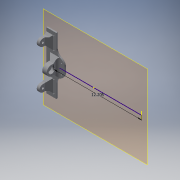
# Autodesk Inventor part: YEnd
Saved by Autodesk Inventor 2016 (Build 200138000, 138)
## iProperties
Created: 2016-04-23
Part Number: YEnd
Material: Generic
Document SubType Name: Modeling
Designer: Scott
Density: 1 g/cm^3
Appearance: Default
Author: Scott
Autodesk Inventor part; units mm, degrees
ref_plane "YZ Plane" through (0, 0, 0) normal (1, 0, 0) x (0, 1, 0)
ref_plane "XZ Plane" through (0, 0, 0) normal (0, 1, 0) x (-1, 0, 0)
ref_plane "XY Plane" through (0, 0, 0) normal (0, 0, 1) x (1, 0, 0)
ref_plane "Work Plane1" through (0, 0, 0) normal (0, 0, 1) x (1, 0, 0)
sketch "Sketch1" plane through (0, 0, 0) normal (0, 0, 1) x (1, 0, 0)
  circle A0 centre (-142.875, 44.45) radius 2.2225
  circle A1 centre (-142.875, 88.9) radius 2.2225
  circle A2 centre (-115.9342, 17.5092) radius 2.2225
  circle A3 centre (-115.9342, -17.5092) radius 2.2225
  circle A4 centre (-142.875, -44.45) radius 2.2225
  circle A5 centre (-142.875, -88.9) radius 2.2225
  line L0 (-168.275, 133.904) -> (-168.275, -133.904)
  line L1 (-103.6936, -28.7748) -> (-168.275, -28.7748)
  line L2 (-168.275, -28.7748) -> (-168.275, 28.7748)
  line L3 (-168.275, 28.7748) -> (-103.6936, 28.7748)
  line L4 (-103.6936, 28.7748) -> (-103.6936, -28.7748)
  line L5 (-103.6936, -28.7748) -> (-168.275, 28.7748) construction
  line L6 (-168.275, -28.7748) -> (-103.6936, 28.7748) construction
  line L7 (-133.3967, -101.2471) -> (-168.275, -101.2471)
  line L8 (-168.275, -101.2471) -> (-168.275, 101.2471)
  line L9 (-168.275, 101.2471) -> (-133.3967, 101.2471)
  line L10 (-133.3967, 101.2471) -> (-133.3967, -101.2471)
  line L11 (-133.3967, -101.2471) -> (-168.275, 101.2471) construction
  line L12 (-168.275, -101.2471) -> (-133.3967, 101.2471) construction
  point P0 (0, 0)
  point P1 (-135.9843, 0)
  point P2 (-150.8358, 0)
extrude "Extrusion1" add sketch "Sketch1" along normal blind 5.08
fillet "Fillet1" radius 25.4 4 edges at (-133.3967, 28.7748, 2.54) (-133.3967, -28.7748, 2.54) (-103.6936, 28.7748, 2.54) (-103.6936, -28.7748, 2.54)
sketch "Sketch2" plane through (0, 0, 5.08) normal (0, 0, 1) x (1, 0, 0)
  line L0 (168.275, 12.5) -> (168.275, -12.5) projected
  line L1 (168.275, 0) -> (-141.725, 0)
  point P0 (0, 0)
  dimension "d3" = 310
  constraints: 2 end point, 1 horizontal, 1 midpoint
  measures "d3" distance of L1.start L1.end
ref_plane "Work Plane2" through (-141.725, 0, 5.08) normal (-1, 0, 0) x (0, -1, 0)
sketch "Sketch3" plane through (-141.725, 0, 5.08) normal (-1, 0, 0) x (0, -1, 0)
  circle A0 centre (0, 21.59) radius 5 projected
  circle A1 centre (0, 21.59) radius 11 projected
  circle A2 centre (0, 21.59) radius 17.3577
  line L0 (-17.3577, 21.59) -> (-17.3577, 0)
  line L1 (-101.2471, 0) -> (101.2471, 0) projected
  line L2 (17.3577, 21.59) -> (17.3577, 0)
  circle A3 centre (-70, 21.59) radius 4 projected
  circle A4 centre (70, 21.59) radius 4 projected
  circle A5 centre (-70, 21.59) radius 12.7105
  circle A6 centre (70, 21.59) radius 12.7105
  line L3 (82.7105, 21.59) -> (82.7105, 0)
  line L4 (57.2895, 21.59) -> (57.2895, 0)
  line L5 (-57.2895, 21.59) -> (-57.2895, 0)
  line L6 (-82.7105, 21.59) -> (-82.7105, 0)
  line L7 (-82.7105, 0) -> (-57.2895, 0)
  line L8 (-17.3577, 0) -> (17.3577, 0)
  line L9 (57.2895, 0) -> (82.7105, 0)
  point P0 (0, -5.08)
  constraints: 18 end point, 6 perpendicular, 6 point on circle, 6 point on line, 5 tangent, 3 centre point, 3 coincident, 1 collinear, 1 parallel, 1 vertical
extrude "Extrusion2" add sketch "Sketch3" against normal up to surface (8.3283 mm away) contours A2 | L2 L1 L0 A2 | L6 A5 L5 L1 | A5 | L4 A6 L3 L1 | A6
sketch "Sketch4" plane through (-141.725, 0, 5.08) normal (-1, 0, 0) x (0, 0, 1)
  circle A0 centre (21.59, 70) radius 4 projected
  line L0 (0, 57.2895) -> (21.59, 57.2895) projected
  arc A1 (21.59, 57.2895) -> (21.59, 82.7105) centre (21.59, 70) ccw projected
  line L1 (21.59, 82.7105) -> (0, 82.7105) projected
  line L2 (0, 57.2895) -> (0, 82.7105) projected
  circle A2 centre (21.59, -70) radius 4 projected
  line L3 (0, -82.7105) -> (0, -57.2895) projected
  line L4 (0, -82.7105) -> (21.59, -82.7105) projected
  arc A3 (21.59, -82.7105) -> (21.59, -57.2895) centre (21.59, -70) ccw projected
  line L5 (21.59, -57.2895) -> (0, -57.2895) projected
  point P0 (-5.08, 0)
extrude "Extrusion3" add sketch "Sketch4" along normal blind 10.16
chamfer "Chamfer1" distance 14.2875 angle 45 2 edges at (-151.885, 70, 5.08) (-151.885, -70, 5.08)
sketch "Sketch5" plane through (-133.3967, -17.3577, 5.08) normal (1, 0, 0) x (0, 0, -1)
  line L0 (0, 34.7154) -> (0, 0) projected
  line L1 (-21.59, 34.7154) -> (0, 34.7154) projected
  arc A0 (-21.59, 34.7154) -> (-21.59, 0) centre (-21.59, 17.3577) ccw projected
  line L2 (0, 0) -> (-21.59, 0) projected
  circle A1 centre (-21.59, 17.3577) radius 11 projected
  circle A2 centre (-21.59, 17.3577) radius 5
  point P0 (5.08, 17.3577)
  dimension "d11" = 10
  constraints: 1 centre point, 1 coincident
  measures "d11" diameter of A2
extrude "Extrusion4" add sketch "Sketch5" along normal blind 5.08 contours L0 L2 A0 L1 | A1
fillet "Fillet2" radius 9.525 1 edges at (-128.3167, 0, 5.08)
chamfer "Chamfer2" distance 14.2875 angle 45 1 edges at (-141.725, 0, 5.08)
sketch "Sketch6" plane through (-133.3967, -101.2471, 5.08) normal (1, 0, 0) x (0, 0, -1)
  line L0 (0, 18.5366) -> (-14.2875, 18.5366) projected
  line L1 (-14.2875, 18.5366) -> (-14.2875, 43.9576) projected
  line L2 (-14.2875, 43.9576) -> (0, 43.9576) projected
  line L3 (0, 43.9576) -> (0, 18.5366) projected
  line L4 (-14.2875, 18.5366) -> (-14.2875, 43.9576) projected
  line L5 (-14.2875, 18.5366) -> (-21.59, 18.5366) projected
  arc A0 (-21.59, 43.9576) -> (-21.59, 18.5366) centre (-21.59, 31.2471) ccw projected
  line L6 (-21.59, 43.9576) -> (-14.2875, 43.9576) projected
  circle A1 centre (-21.59, 31.2471) radius 4 projected
  line L7 (-14.2875, 158.5366) -> (-14.2875, 183.9576) projected
  line L8 (-14.2875, 158.5366) -> (-21.59, 158.5366) projected
  arc A2 (-21.59, 183.9576) -> (-21.59, 158.5366) centre (-21.59, 171.2471) ccw projected
  line L9 (-21.59, 183.9576) -> (-14.2875, 183.9576) projected
  circle A3 centre (-21.59, 171.2471) radius 4 projected
  line L10 (0, 158.5366) -> (-14.2875, 158.5366) projected
  line L11 (-14.2875, 158.5366) -> (-14.2875, 183.9576) projected
  line L12 (-14.2875, 183.9576) -> (0, 183.9576) projected
  line L13 (0, 183.9576) -> (0, 158.5366) projected
  point P0 (5.08, 101.2471)
extrude "Extrusion5" add sketch "Sketch6" against normal up to surface (34.8783 mm away) contours L0 L1 L2 L3 | L5 A0 L6 L1 | A1 | L8 A2 L9 L7 | L7 L12 L13 L10
sketch "Sketch7" plane through (-133.3967, 101.2471, 5.08) normal (1, 0, 0) x (0, 0, -1)
  circle A0 centre (-21.59, -31.2471) radius 4 projected
  line L0 (5.08, 0) -> (5.08, -202.4943) projected
  line L1 (5.08, -202.4943) -> (0, -202.4943) projected
  line L2 (0, -183.9576) -> (0, -202.4943) projected
  line L3 (-21.59, -183.9576) -> (0, -183.9576) projected
  arc A1 (-21.59, -158.5366) -> (-21.59, -183.9576) centre (-21.59, -171.2471) ccw projected
  line L4 (0, -158.5366) -> (-21.59, -158.5366) projected
  line L5 (0, -43.9576) -> (0, -158.5366) projected
  line L6 (-21.59, -43.9576) -> (0, -43.9576) projected
  arc A2 (-21.59, -18.5366) -> (-21.59, -43.9576) centre (-21.59, -31.2471) ccw projected
  line L7 (0, -18.5366) -> (-21.59, -18.5366) projected
  line L8 (0, 0) -> (0, -18.5366) projected
  line L9 (5.08, 0) -> (0, 0) projected
  line L10 (0, -18.5366) -> (0, -43.9576)
  line L11 (0, -132.3159) -> (0, -155.422) projected
  line L12 (0, -155.422) -> (0, -183.9576)
  line L13 (0, -192.3696) -> (0, -187.9246) projected
  point P0 (5.08, -101.2471)
  constraints: 4 end point, 1 collinear, 1 vertical
extrude "Extrusion6" cut sketch "Sketch7" against normal blind 25.4 contours L10 L6 A2 L7 | L3 A1 L4 L12
chamfer "Chamfer3" distance 14.2875 angle 45 2 edges at (-158.7967, 70, 5.08) (-158.7967, -70, 5.08)
chamfer "Chamfer4" distance 14.2875 angle 45 6 edges at (-151.6529, 57.2895, 5.08) (-163.5358, 57.2895, 5.08) (-163.5358, -57.2895, 5.08) (-151.6529, -57.2895, 5.08) (-137.4021, 17.3577, 5.08) (-137.4021, -17.3577, 5.08)
chamfer "Chamfer5" distance 6.35 angle 45 2 edges at (-156.3921, -82.7105, 5.08) (-156.3921, 82.7105, 5.08)
sketch "Sketch8" plane through (-168.275, -101.2471, 0) normal (-1, 0, 0) x (0, 0, 1)
  circle A0 centre (26.67, 31.2471) radius 4 projected
  point P0 (0, 101.2471)
extrude "Extrusion7" cut sketch "Sketch8" against normal blind 25.4
sketch "Sketch9" plane through (-141.725, 0, 5.08) normal (-1, 0, 0) x (0, 0, 1)
  circle A0 centre (21.59, 0) radius 5 projected
  circle A1 centre (21.59, 0) radius 11 projected
  point P0 (-5.08, 0)
extrude "Extrusion8" add sketch "Sketch9" against normal blind 2
sketch "Sketch10" plane through (-139.725, 0, 26.67) normal (1, 0, 0) x (0, 0, -1)
  circle A0 centre (0, 0) radius 11 projected
  point P0 (26.67, 0)
extrude "Extrusion9" cut sketch "Sketch10" along normal blind 37.6875
sketch "Sketch11" plane through (-141.725, 0, 5.08) normal (-1, 0, 0) x (0, 0, 1)
  circle A0 centre (21.59, 0) radius 5 projected
  line L0 (14.2875, 8.2264) -> (14.2875, 17.3577) projected
  arc A1 (14.2875, 8.2264) -> (14.2875, -8.2264) centre (21.59, 0) ccw projected
  line L1 (14.2875, -17.3577) -> (14.2875, -8.2264) projected
  line L2 (14.2875, -17.3577) -> (21.59, -17.3577) projected
  arc A2 (21.59, -17.3577) -> (21.59, 17.3577) centre (21.59, 0) ccw projected
  line L3 (21.59, 17.3577) -> (14.2875, 17.3577) projected
  line L4 (14.2875, 8.2264) -> (14.2875, 17.3577) projected
  line L5 (6.8925, -17.3577) -> (14.2875, -17.3577)
  line L6 (14.2875, -17.3577) -> (14.2875, 17.3577)
  line L7 (14.2875, 17.3577) -> (6.8925, 17.3577)
  line L8 (6.8925, 17.3577) -> (6.8925, -17.3577)
  line L9 (6.8925, -17.3577) -> (14.2875, 17.3577) construction
  line L10 (14.2875, -17.3577) -> (6.8925, 17.3577) construction
  point P0 (-5.08, 0)
  point P1 (10.59, 0)
  constraints: 12 end point, 2 midpoint, 2 parallel, 1 horizontal, 1 perpendicular, 1 point on circle
extrude "Extrusion10" add sketch "Sketch11" along normal blind 2.54
body "Solid1"
